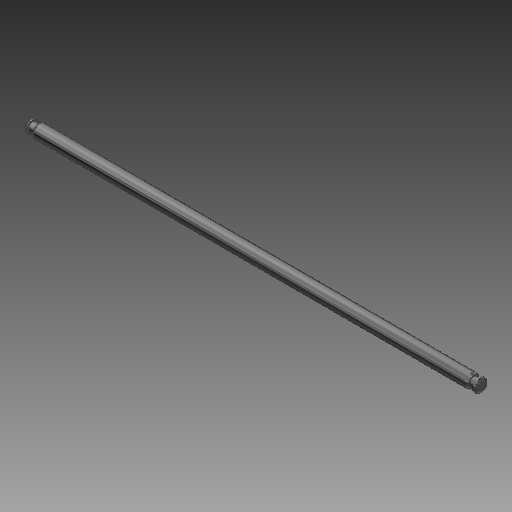
# Autodesk Inventor part: 311-03
Saved by Autodesk Inventor 2019 (Build 230136000, 136)
## iProperties
Company: Autodesk Inc.
Created: 2007-10-25
Part Number: 311-03
Document SubType Name: Modeling
Designer: Autodesk Inc.
Density: 7.85 g/cm^3
Mass: 343.054 g
Surface Area: 150.138 cm^2
Volume: 43.7011 cm^3
Material: Steel
Description: SUPPORT ROD
Appearance: Rubber - Black - Version 1.1
Component Category: Lower Component
Author: Inventor
Autodesk Inventor part; units mm, degrees
note: some values were not read from the file. Chosen so that the rebuilt part matches the saved one: edges of "Fillet1".
ref_plane "YZ Plane" through (0, 0, 0) normal (1, 0, 0) x (0, 1, 0)
ref_plane "XZ Plane" through (0, 0, 0) normal (0, 1, 0) x (-1, 0, 0)
sketch "Sketch1" plane through (0, 0, 0) normal (0, 0, 1) x (1, 0, 0)
  line L0 (196.45, 0) -> (-196.45, 0)
  line L1 (-196.45, 0) -> (-196.45, 3.125)
  line L2 (-193.575, 6) -> (-193.5, 6)
  line L3 (-193.5, 6) -> (-193.5, 4)
  line L4 (-193.5, 4) -> (-189, 4)
  line L5 (-189, 4) -> (-189, 6)
  line L6 (-189, 6) -> (189, 6)
  line L7 (189, 6) -> (189, 4)
  line L8 (189, 4) -> (193.5, 4)
  line L9 (193.5, 4) -> (193.5, 6)
  line L10 (193.5, 6) -> (193.575, 6)
  line L11 (196.45, 3.125) -> (196.45, 0)
  arc A0 (-193.575, 6) -> (-196.45, 3.125) centre (-193.575, 3.125) ccw
  arc A1 (196.45, 3.125) -> (193.575, 6) centre (193.575, 3.125) ccw
  point P0 (0, 0)
  point P1 (0, 0)
  dimension "d2" = 12
  dimension "d4" = 8
  dimension "d5" = 12
  dimension "d7" = 8
  dimension "d8" = 12
  dimension "d15" = 2.875
  dimension "d21" = 2.95
  dimension "d22" = 4.5
  dimension "d23" = 2.95
  dimension "d24" = 4.5
  dimension "d29" = 387
  constraints: 24 end point, 7 parallel, 4 point on circle, 4 tangent, 2 centre point, 2 collinear, 2 perpendicular, 1 coincident, 1 equal radius, 1 horizontal, 1 midpoint
  measures "d2" diameter of L6 L0
  measures "d4" diameter of L4 L0
  measures "d5" diameter of L2 L0
  measures "d7" diameter of L8 L0
  measures "d8" diameter of L10 L0
  measures "d15" radius of A0
  measures "d21" distance between parallel lines of L3 L1
  measures "d22" distance of L3.end L4.end
  measures "d23" distance between parallel lines of L9 L11
  measures "d24" distance of L7.end L8.end
  measures "d29" distance between parallel lines of L9 L3
revolve "Revolution1" add sketch "Sketch1" angle 360 about axis through (196.45, 0, 0) along (-1, 0, 0)
chamfer "Chamfer1" distance 2 angle 20 1 edges at (-189, -6, 0) measured on face at (-63, 5.9223, 0.9625)
fillet "Fillet1" radius 0.5 2 edges at (189, -4, 0) (-189, -4, 0)
chamfer "Chamfer2" distance 2 angle 20 1 edges at (189, -6, 0) measured on face at (-61.6667, 5.9805, 0.4828)
ref_plane "Work Plane1" through (-81.95, 0, 0) normal (-1, 0, 0) x (0, 0, 1)
split_face "Split1"
equation "\"d2\" = d5"
equation "\"d7\" = d4"
equation "\"d8\" = d5"
equation "\"d24\" = d22"
body "Solid1"
